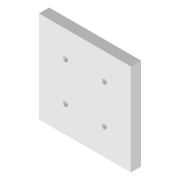
# Autodesk Inventor part: Sujeción Cilindro Cortadora
Saved by Autodesk Inventor 2021 (Build 250183000, 183)
## iProperties
Created: 2021-08-11
Part Number: Sujeción Cilindro Cortadora
Material: Generic
Document SubType Name: Modeling
Designer: maaro
Density: 1 g/cm^3
Appearance: Default
Author: maaro
Autodesk Inventor part; units mm, degrees
ref_plane "YZ Plane" through (0, 0, 0) normal (1, 0, 0) x (0, 1, 0)
ref_plane "XZ Plane" through (0, 0, 0) normal (0, 1, 0) x (-1, 0, 0)
ref_plane "XY Plane" through (0, 0, 0) normal (0, 0, 1) x (1, 0, 0)
ref_plane "Work Plane1" through (0, 0, 0) normal (0, 0, 1) x (1, 0, 0)
sketch "Sketch1" plane through (0, 0, 0) normal (0, 0, 1) x (1, 0, 0)
  line L0 (45, 45) -> (-45, 45)
  line L1 (-45, 45) -> (-45, -45)
  line L2 (-45, -45) -> (45, -45)
  line L3 (45, -45) -> (45, 45)
  line L4 (45, 45) -> (-45, -45) construction
  line L5 (-45, 45) -> (45, -45) construction
  circle A0 centre (19, 19) radius 2.4585 projected
  circle A1 centre (19, -19) radius 2.4585 projected
  circle A2 centre (-19, -19) radius 2.4585 projected
  circle A3 centre (-19, 19) radius 2.4585 projected
  point P0 (0, 0)
  point P1 (0, 0)
  dimension "d0" = 90
  dimension "d1" = 90
  constraints: 12 end point, 2 parallel, 2 perpendicular, 1 coincident, 1 horizontal, 1 midpoint, 1 point on line
  measures "d0" distance of L1.end L2.end
  measures "d1" distance of L0.end L1.end
extrude "Extrusion1" add sketch "Sketch1" along normal blind 10
body "Solid1"
